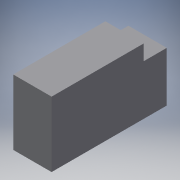
# Autodesk Inventor part: CNC
Saved by Autodesk Inventor 2019.4 (Build 234330000, 330)
## iProperties
Created: 2019-10-31
Part Number: CNC
Material: Generic
Document SubType Name: Modeling
Designer: holecep
Density: 1 g/cm^3
Appearance: Default
Author: holecep
Autodesk Inventor part; units mm, degrees
ref_plane "YZ Plane" through (0, 0, 0) normal (1, 0, 0) x (0, 1, 0)
ref_plane "XZ Plane" through (0, 0, 0) normal (0, 1, 0) x (-1, 0, 0)
ref_plane "XY Plane" through (0, 0, 0) normal (0, 0, 1) x (1, 0, 0)
sketch "Sketch1" plane through (0, 0, 0) normal (0, 1, 0) x (-1, 0, 0)
  line L0 (0, 0) -> (1270, 0)
  line L1 (1270, 0) -> (1270, -3810)
  line L2 (1270, -3810) -> (0, -3810)
  line L3 (0, -3810) -> (0, 0)
  dimension "d0" = 3810
  dimension "d1" = 1270
  constraints: 8 end point, 2 parallel, 1 horizontal, 1 perpendicular
  measures "d0" distance of L2.end L0.start
  measures "d1" distance of L0.start L0.end
extrude "Extrusion1" add sketch "Sketch1" along normal blind 2159
sketch "Sketch2" plane through (0, 2159, 0) normal (0, 1, 0) x (1, 0, 0)
  line L0 (0, 0) -> (0, 3810) projected
  line L1 (0, 3810) -> (-1270, 3810) projected
  line L2 (-1270, 3810) -> (-1270, 0) projected
  line L3 (-1270, 3048) -> (0, 3048)
  dimension "d5" = 762
  constraints: 2 end point, 2 point on line, 1 horizontal
  measures "d5" distance between parallel lines of L1 L3
extrude "Extrusion2" cut sketch "Sketch2" against normal blind 508
body "Solid1"
